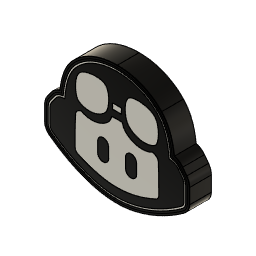
copilot-lamp (Autodesk Fusion 360 design; units mm, degrees)
Autodesk Fusion 360 part; units mm, degrees
sketch "Sketch1" plane through (0, 0, 0) normal (0, 1, 0) x (1, 0, 0)
  line L0 (0, 0) -> (250, 0)
  line L1 (250, 0) -> (250, 250)
  line L2 (250, 250) -> (0, 250)
  line L3 (0, 250) -> (0, 0)
  line L4 (10, 10) -> (240, 10)
  line L5 (240, 10) -> (240, 240)
  line L6 (240, 240) -> (10, 240)
  line L7 (10, 240) -> (10, 10)
  dimension "d1" = 250
  dimension "d2" = 250
  dimension "d3" = -10
  constraint horizontal L0
  constraint vertical L1
  constraint horizontal L2
  constraint vertical L3
  constraint coincident L0.start L3.end
  measures "d1" distance of L0.start L0.end
  measures "d2" distance of L0.start L2.end
sketch "Sketch2" plane through (0, 0, 0) normal (0, 1, 0) x (1, 0, 0)
  spline S0 degree 3 poles (158.5521, 137.3198) (158.5521, 132.1805) (154.3858, 128.0143) (149.2467, 128.0143) knots 0 0 0 0 1 1 1 1
  spline S1 degree 3 poles (149.2467, 128.0143) (144.1075, 128.0143) (139.9413, 132.1805) (139.9413, 137.3198) knots 0 0 0 0 1 1 1 1
  line L0 (139.9413, 137.3198) -> (139.9413, 154.4712)
  spline S2 degree 3 poles (139.9413, 154.4712) (139.9413, 159.6094) (144.1075, 163.7764) (149.2467, 163.7764) knots 0 0 0 0 1 1 1 1
  spline S3 degree 3 poles (149.2467, 163.7764) (154.3858, 163.7764) (158.5521, 159.6094) (158.5521, 154.4712) knots 0 0 0 0 1 1 1 1
  line L1 (158.5521, 154.4712) -> (158.5521, 137.3198)
  spline S4 degree 3 poles (101.5644, 128.0143) (106.7036, 128.0143) (110.8699, 132.1805) (110.8699, 137.3198) knots 0 0 0 0 1 1 1 1
  line L2 (110.8699, 137.3198) -> (110.8699, 154.4712)
  spline S5 degree 3 poles (110.8699, 154.4712) (110.8699, 159.6094) (106.7036, 163.7764) (101.5644, 163.7764) knots 0 0 0 0 1 1 1 1
  spline S6 degree 3 poles (101.5644, 163.7764) (96.425, 163.7764) (92.2595, 159.6094) (92.2595, 154.4712) knots 0 0 0 0 1 1 1 1
  line L3 (92.2595, 154.4712) -> (92.2595, 137.3198)
  spline S7 degree 3 poles (92.2595, 137.3198) (92.2595, 132.1805) (96.425, 128.0143) (101.5644, 128.0143) knots 0 0 0 0 1 1 1 1
  line L4 (10.7372, 128.4911) -> (10.7372, 154.1394)
  spline S8 degree 3 poles (10.7372, 154.1394) (10.7429, 157.4509) (12.3851, 160.6794) (15.0572, 162.6363) knots 0 0 0 0 1 1 1 1
  spline S9 degree 3 poles (15.0572, 162.6363) (46.6019, 185.7298) (85.5234, 204.3058) (125.1746, 204.3058) knots 0 0 0 0 1 1 1 1
  spline S10 degree 3 poles (125.1746, 204.3058) (169.0412, 204.3058) (212.9606, 179.028) (235.2919, 162.6363) knots 0 0 0 0 1 1 1 1
  spline S11 degree 3 poles (235.2919, 162.6363) (237.9639, 160.6794) (239.6054, 157.4509) (239.6119, 154.1394) knots 0 0 0 0 1 1 1 1
  line L5 (239.6119, 154.1394) -> (239.6119, 128.4911)
  spline S12 degree 3 poles (239.6119, 128.4911) (239.6119, 125.1152) (238.539, 121.8537) (236.5507, 119.1358) knots 0 0 0 0 1 1 1 1
  line L6 (236.5507, 119.1358) -> (229.5843, 109.7091)
  spline S13 degree 3 poles (229.5843, 109.7091) (225.8533, 104.6514) (220.3047, 103.3149) (214.3928, 103.3149) knots 0 0 0 0 1 1 1 1
  spline S14 degree 3 poles (214.3928, 103.3149) (212.1612, 77.8526) (206.8828, 59.6856) (194.2661, 46.3823) knots 0 0 0 0 1 1 1 1
  spline S15 degree 3 poles (194.2661, 46.3823) (170.2343, 20.92) (138.3348, 18.3452) (125.1746, 18.3452) knots 0 0 0 0 1 1 1 1
  spline S16 degree 3 poles (125.1746, 18.3452) (112.0143, 18.3452) (80.1149, 20.92) (56.083, 46.3823) knots 0 0 0 0 1 1 1 1
  spline S17 degree 3 poles (56.083, 46.3823) (43.4806, 59.6856) (38.1879, 77.8526) (35.9563, 103.3149) knots 0 0 0 0 1 1 1 1
  spline S18 degree 3 poles (35.9563, 103.3149) (30.0328, 103.3149) (24.5083, 104.6285) (20.7791, 109.7091) knots 0 0 0 0 1 1 1 1
  line L7 (20.7791, 109.7091) -> (13.8127, 119.1501)
  spline S19 degree 3 poles (13.8127, 119.1501) (11.8101, 121.868) (10.7372, 125.1152) (10.7372, 128.4911) knots 0 0 0 0 1 1 1 1
  spline S20 degree 3 poles (54.3951, 116.8328) (54.7012, 110.991) (59.4446, 108.6987) (64.3797, 107.077) knots 0 0 0 0 1 1 1 1
  spline S21 degree 3 poles (64.3797, 107.077) (69.5838, 110.3418) (75.9379, 111.6259) (82.0174, 111.6259) knots 0 0 0 0 1 1 1 1
  spline S22 degree 3 poles (82.0174, 111.6259) (88.4831, 111.6259) (100.5419, 110.081) (110.5695, 100.0677) knots 0 0 0 0 1 1 1 1
  spline S23 degree 3 poles (110.5695, 100.0677) (113.1014, 97.5501) (114.8323, 93.602) (116.0053, 89.2248) knots 0 0 0 0 1 1 1 1
  spline S24 degree 3 poles (116.0053, 89.2248) (119.0474, 88.9154) (122.1026, 88.7532) (125.1602, 88.7384) knots 0 0 0 0 1 1 1 1
  spline S25 degree 3 poles (125.1602, 88.7384) (127.8781, 88.7384) (131.0109, 88.8958) (134.3438, 89.2248) knots 0 0 0 0 1 1 1 1
  spline S26 degree 3 poles (134.3438, 89.2248) (135.5168, 93.602) (137.2477, 97.5501) (139.7796, 100.0677) knots 0 0 0 0 1 1 1 1
  spline S27 degree 3 poles (139.7796, 100.0677) (149.7929, 110.081) (161.866, 111.6259) (168.3317, 111.6259) knots 0 0 0 0 1 1 1 1
  spline S28 degree 3 poles (168.3317, 111.6259) (174.4131, 111.6259) (180.7835, 110.3561) (185.9837, 107.077) knots 0 0 0 0 1 1 1 1
  spline S29 degree 3 poles (185.9837, 107.077) (190.9031, 108.6934) (195.6269, 111.0244) (195.9397, 116.8328) knots 0 0 0 0 1 1 1 1
  spline S30 degree 3 poles (195.9397, 116.8328) (196.4636, 127.812) (196.5091, 138.7809) (196.5545, 149.755) knots 0 0 0 0 1 1 1 1
  spline S31 degree 3 poles (196.5545, 149.755) (196.5774, 155.2623) (196.6002, 160.771) (196.6836, 166.284) knots 0 0 0 0 1 1 1 1
  spline S32 degree 3 poles (196.6836, 166.284) (196.6614, 169.484) (194.7328, 172.455) (191.82, 173.7797) knots 0 0 0 0 1 1 1 1
  spline S33 degree 3 poles (191.82, 173.7797) (168.1458, 184.5654) (145.759, 190.0011) (125.1602, 190.0011) knots 0 0 0 0 1 1 1 1
  spline S34 degree 3 poles (125.1602, 190.0011) (104.5901, 190.0011) (82.2033, 184.5654) (58.5434, 173.7797) knots 0 0 0 0 1 1 1 1
  spline S35 degree 3 poles (58.5434, 173.7797) (55.631, 172.455) (53.7013, 169.484) (53.6798, 166.284) knots 0 0 0 0 1 1 1 1
  spline S36 degree 3 poles (53.6798, 166.284) (53.3966, 149.8179) (53.624, 133.2834) (54.4094, 116.8328) knots 0 0 0 0 1 1 1 1
  line L8 (54.4094, 116.8328) -> (54.3951, 116.8328)
  spline S37 degree 3 poles (191.5482, 93.8738) (187.6859, 97.7361) (180.3906, 100.3109) (172.523, 100.3109) knots 0 0 0 0 1 1 1 1
  spline S38 degree 3 poles (172.523, 100.3109) (166.515, 100.3109) (155.0713, 99.0235) (145.6302, 89.4393) knots 0 0 0 0 1 1 1 1
  spline S39 degree 3 poles (145.6302, 89.4393) (141.4819, 85.434) (138.907, 75.4208) (139.1931, 65.2645) knots 0 0 0 0 1 1 1 1
  spline S40 degree 3 poles (139.1931, 65.2645) (139.4792, 57.1108) (141.768, 50.3876) (145.2011, 47.5267) knots 0 0 0 0 1 1 1 1
  spline S41 degree 3 poles (145.2011, 47.5267) (148.9203, 44.2366) (157.3601, 42.8061) (166.8011, 43.6644) knots 0 0 0 0 1 1 1 1
  spline S42 degree 3 poles (166.8011, 43.6644) (176.8144, 44.6657) (185.2541, 47.9558) (189.5455, 52.5333) knots 0 0 0 0 1 1 1 1
  spline S43 degree 3 poles (189.5455, 52.5333) (198.8436, 62.6896) (196.8409, 88.438) (191.5482, 93.8738) knots 0 0 0 0 1 1 1 1
  spline S44 degree 3 poles (133.1852, 68.8406) (132.8991, 70.4141) (132.756, 72.1307) (132.613, 73.9903) knots 0 0 0 0 1 1 1 1
  spline S45 degree 3 poles (132.613, 73.9903) (132.613, 75.2777) (132.613, 76.5651) (132.756, 77.9956) knots 0 0 0 0 1 1 1 1
  spline S46 degree 3 poles (132.756, 77.9956) (129.8951, 77.7095) (127.4633, 77.7095) (125.1746, 77.7095) knots 0 0 0 0 1 1 1 1
  spline S47 degree 3 poles (125.1746, 77.7095) (122.8861, 77.7095) (120.454, 77.7095) (117.5931, 77.9956) knots 0 0 0 0 1 1 1 1
  spline S48 degree 3 poles (117.5931, 77.9956) (117.7361, 76.5651) (117.7361, 75.278) (117.7361, 73.9906) knots 0 0 0 0 1 1 1 1
  spline S49 degree 3 poles (117.7361, 73.9906) (117.5931, 72.131) (117.45, 70.4141) (117.1639, 68.8406) knots 0 0 0 0 1 1 1 1
  spline S50 degree 3 poles (117.1639, 68.8406) (120.1679, 68.5545) (122.8858, 68.4115) (125.1746, 68.4115) knots 0 0 0 0 1 1 1 1
  spline S51 degree 3 poles (125.1746, 68.4115) (127.4633, 68.4115) (130.1812, 68.5545) (133.1852, 68.8406) knots 0 0 0 0 1 1 1 1
  spline S52 degree 3 poles (111.156, 65.2645) (111.4421, 75.4208) (108.8672, 85.434) (104.7189, 89.4393) knots 0 0 0 0 1 1 1 1
  spline S53 degree 3 poles (104.7189, 89.4393) (95.2778, 99.0235) (83.8341, 100.3109) (77.8261, 100.3109) knots 0 0 0 0 1 1 1 1
  spline S54 degree 3 poles (77.8261, 100.3109) (69.9585, 100.3109) (62.6632, 97.7361) (58.8009, 93.8738) knots 0 0 0 0 1 1 1 1
  spline S55 degree 3 poles (58.8009, 93.8738) (53.5082, 88.438) (51.5055, 62.6896) (60.8036, 52.5333) knots 0 0 0 0 1 1 1 1
  spline S56 degree 3 poles (60.8036, 52.5333) (65.095, 47.9558) (73.5347, 44.6657) (83.548, 43.6644) knots 0 0 0 0 1 1 1 1
  spline S57 degree 3 poles (83.548, 43.6644) (92.9891, 42.8061) (101.4288, 44.2366) (105.148, 47.5267) knots 0 0 0 0 1 1 1 1
  spline S58 degree 3 poles (105.148, 47.5267) (108.5811, 50.3876) (110.8699, 57.1108) (111.156, 65.2645) knots 0 0 0 0 1 1 1 1
  line L9 (7.7372, 128.4911) -> (7.7372, 154.1445)
  spline S59 degree 3 poles (7.7372, 154.1445) (7.7441, 158.1057) (9.5073, 161.8673) (12.4918, 164.4276) (12.747, 164.6466) (13.0114, 164.8566) (13.2847, 165.0567) (13.2848, 165.0567) (13.2848, 165.0568) (13.2849, 165.0568) knots 0 0 0 0 0.921211 0.921211 0.921211 1 1 1 1.000024 1.000024 1.000024 1.000024
  spline S60 degree 3 poles (13.2849, 165.0568) (13.285, 165.0569) (13.285, 165.0569) (13.2851, 165.057) (38.021, 183.1658) (67.2869, 198.586) (98.1418, 204.6126) (107.0469, 206.352) (116.084, 207.3058) (125.1746, 207.3058) knots -0.000002 -0.000002 -0.000002 -0.000002 0 0 0 0.776029 0.776029 0.776029 1 1 1 1
  spline S61 degree 3 poles (125.1746, 207.3058) (151.1392, 207.3058) (176.8345, 198.726) (198.2832, 188.335) (214.0222, 180.7101) (227.4746, 172.0956) (237.0644, 165.0567) knots 0 0 0 0 0.576746 0.576746 0.576746 0.999961 0.999961 0.999961 0.999961
  spline S62 degree 3 poles (237.0644, 165.0567) (240.2611, 162.7155) (242.2626, 159.0731) (242.5713, 155.1511) (242.5975, 154.8176) (242.6112, 154.4821) (242.6119, 154.1452) (242.6119, 154.1442) (242.6119, 154.1433) (242.6119, 154.1423) knots 0 0 0 0 0.92164 0.92164 0.92164 1 1 1 1.000295 1.000295 1.000295 1.000295
  line L10 (242.6119, 154.1423) -> (242.6119, 128.4911)
  spline S63 degree 3 poles (242.6119, 128.4911) (242.6119, 124.4796) (241.3319, 120.5904) (238.9719, 117.3645) (238.9705, 117.3626) (238.9691, 117.3606) (238.9677, 117.3587) knots 0 0 0 0 1 1 1 1.000715 1.000715 1.000715 1.000715
  line L11 (238.9677, 117.3587) -> (231.9977, 107.9271)
  spline S64 degree 3 poles (231.9977, 107.9271) (229.8034, 104.953) (226.9585, 102.9755) (223.9284, 101.8321) (221.7257, 101.0009) (219.4347, 100.5852) (217.1364, 100.413) knots 0.000057 0.000057 0.000057 0.000057 0.495955 0.495955 0.495955 0.856432 0.856432 0.856432 0.856432
  spline S65 degree 3 poles (217.1364, 100.413) (215.652, 85.2695) (213.0029, 72.5806) (208.1192, 61.8381) (205.1344, 55.2727) (201.3057, 49.4466) (196.4478, 44.3231) knots 0.034498 0.034498 0.034498 0.034498 0.633678 0.633678 0.633678 0.999875 0.999875 0.999875 0.999875
  spline S66 degree 3 poles (196.4478, 44.3232) (182.9181, 29.9881) (166.9642, 22.6605) (153.1177, 18.9787) (141.5097, 15.8921) (131.3545, 15.3452) (125.1746, 15.3452) knots 0 0 0 0 0.543971 0.543971 0.543971 1 1 1 1
  spline S67 degree 3 poles (125.1746, 15.3452) (116.3753, 15.3452) (99.5093, 16.4426) (81.8828, 24.4301) (72.3644, 28.7433) (62.6264, 35.0798) (53.9051, 44.3191) knots 0 0 0 0 0.649314 0.649314 0.649314 0.999949 0.999949 0.999949 0.999949
  spline S68 degree 3 poles (53.9051, 44.3191) (46.3224, 52.3236) (41.2686, 62.0288) (37.9494, 73.6262) (35.6681, 81.5973) (34.1875, 90.4726) (33.2128, 100.4115) knots 0 0 0 0 0.572201 0.572201 0.572201 0.965484 0.965484 0.965484 0.965484
  spline S69 degree 3 poles (33.2128, 100.4115) (30.5434, 100.609) (27.8843, 101.1321) (25.3703, 102.2565) (22.7389, 103.4334) (20.2964, 105.2967) (18.3607, 107.9339) knots 0.143547 0.143547 0.143547 0.143547 0.562009 0.562009 0.562009 1 1 1 1
  line L12 (18.3607, 107.9339) -> (11.3976, 117.3705)
  spline S70 degree 3 poles (11.3976, 117.3705) (9.0215, 120.5952) (7.7372, 124.4796) (7.7372, 128.4911) knots 0 0 0 0 1 1 1 1
  spline S71 degree 3 poles (8.9824, 115.5909) (6.233, 119.3223) (4.7372, 123.844) (4.7372, 128.4911) knots 0 0 0 0 1 1 1 1
  line L13 (4.7372, 128.4911) -> (4.7372, 154.1445)
  spline S72 degree 3 poles (4.7372, 154.1445) (4.7372, 154.1463) (4.7372, 154.148) (4.7372, 154.1497) (4.7442, 158.1771) (6.2198, 161.9705) (8.7807, 164.9481) (9.5825, 165.8803) (10.4953, 166.7323) (11.5122, 167.4771) (11.5123, 167.4772) (11.5125, 167.4772) (11.5126, 167.4773) knots -0.000521 -0.000521 -0.000521 -0.000521 0 0 0 0.761555 0.761555 0.761555 1 1 1 1.000048 1.000048 1.000048 1.000048
  spline S73 degree 3 poles (11.5126, 167.4773) (11.5127, 167.4774) (11.5128, 167.4775) (11.513, 167.4776) (32.5289, 182.8631) (56.8066, 196.3546) (82.7045, 203.9271) (96.4932, 207.9589) (110.7471, 210.3058) (125.1746, 210.3058) knots -0.000004 -0.000004 -0.000004 -0.000004 0 0 0 0.65256 0.65256 0.65256 1 1 1 1
  spline S74 degree 3 poles (125.1746, 210.3058) (146.7387, 210.3058) (167.9411, 204.5481) (186.7543, 196.7918) (208.2194, 187.9422) (226.5873, 176.468) (238.837, 167.477) knots 0 0 0 0 0.467044 0.467044 0.467044 0.999924 0.999924 0.999924 0.999924
  spline S75 degree 3 poles (238.837, 167.477) (242.0897, 165.0948) (244.2873, 161.6622) (245.1818, 157.8319) (245.4602, 156.6399) (245.6094, 155.4058) (245.6119, 154.1511) (245.6119, 154.1491) (245.6119, 154.1472) (245.6119, 154.1452) knots 0 0 0 0 0.762657 0.762657 0.762657 1 1 1 1.000589 1.000589 1.000589 1.000589
  line L14 (245.6119, 154.1452) -> (245.6119, 128.4911)
  spline S76 degree 3 poles (245.6119, 128.4911) (245.6119, 123.844) (244.1248, 119.3271) (241.3932, 115.5932) (241.3903, 115.5893) (241.3875, 115.5854) (241.3846, 115.5815) knots 0 0 0 0 1 1 1 1.001431 1.001431 1.001431 1.001431
  line L15 (241.3846, 115.5815) -> (234.4112, 106.1452)
  spline S77 degree 3 poles (234.4112, 106.1452) (232.3088, 103.2959) (229.6221, 101.1651) (226.7745, 99.7909) (224.5136, 98.6997) (222.1772, 98.0622) (219.8733, 97.7062) knots 0.000099 0.000099 0.000099 0.000099 0.410804 0.410804 0.410804 0.736901 0.736901 0.736901 0.736901
  spline S78 degree 3 poles (219.8733, 97.7062) (218.6013, 85.9602) (216.5742, 75.613) (213.2182, 66.4036) (209.8594, 57.1866) (205.124, 49.1134) (198.6246, 42.2588) knots 0.066215 0.066215 0.066215 0.066215 0.532858 0.532858 0.532858 0.99988 0.99988 0.99988 0.99988
  spline S79 degree 3 poles (198.6246, 42.2588) (187.2956, 30.2574) (174.2956, 22.9932) (162.2131, 18.6679) (146.8735, 13.1765) (132.9735, 12.3452) (125.1746, 12.3452) knots 0.000064 0.000064 0.000064 0.000064 0.440648 0.440648 0.440648 1 1 1 1
  spline S80 degree 3 poles (125.1746, 12.3452) (117.5616, 12.3452) (104.1361, 13.1384) (89.2315, 18.2828) (77.5633, 22.31) (64.9648, 29.0431) (53.7854, 40.1449) (53.0936, 40.8319) (52.4073, 41.5355) (51.7272, 42.256) knots 0 0 0 0 0.546006 0.546006 0.546006 0.97345 0.97345 0.97345 0.999902 0.999902 0.999902 0.999902
  line L16 (51.7272, 42.256) -> (51.7196, 42.264)
  spline S81 degree 3 poles (51.7196, 42.264) (45.1771, 49.1727) (40.4206, 57.3182) (37.0555, 66.6268) (33.7472, 75.7787) (31.739, 86.0521) (30.4764, 97.7022) knots 0.000182 0.000182 0.000182 0.000182 0.470924 0.470924 0.470924 0.933737 0.933737 0.933737 0.933737
  spline S82 degree 3 poles (30.4764, 97.7022) (28.8084, 97.9581) (27.1205, 98.3623) (25.4513, 98.9838) (22.5741, 100.0551) (19.7525, 101.8165) (17.4328, 104.3431) (16.9117, 104.9107) (16.4155, 105.5144) (15.947, 106.1522) knots 0.26327 0.26327 0.26327 0.26327 0.5 0.5 0.5 0.908036 0.908036 0.908036 0.999687 0.999687 0.999687 0.999687
  line L17 (15.947, 106.1522) -> (8.9824, 115.5909)
  line L18 (1.7372, 128.4911) -> (1.7372, 154.1471)
  spline S83 degree 3 poles (1.7372, 154.1471) (1.7372, 154.1497) (1.7372, 154.1523) (1.7372, 154.1549) (1.7445, 158.3641) (3.1041, 162.3187) (5.4807, 165.605) (6.6481, 167.2193) (8.0725, 168.6765) (9.7397, 169.8974) (9.7399, 169.8976) (9.7401, 169.8977) (9.7403, 169.8979) knots -0.000782 -0.000782 -0.000782 -0.000782 0 0 0 0.67059 0.67059 0.67059 1 1 1 1.000072 1.000072 1.000072 1.000072
  spline S84 degree 3 poles (9.7403, 169.8979) (9.7405, 169.898) (9.7407, 169.8981) (9.7408, 169.8983) (28.9256, 183.9432) (50.8226, 196.4464) (74.2971, 204.4158) (90.6333, 209.9618) (107.7504, 213.3058) (125.1746, 213.3058) knots -0.000006 -0.000006 -0.000006 -0.000006 0 0 0 0.589654 0.589654 0.589654 1 1 1 1
  spline S85 degree 3 poles (125.1746, 213.3058) (144.9594, 213.3058) (164.3076, 208.5849) (181.8206, 201.9667) (203.0931, 193.9278) (221.6874, 183.0627) (235.0889, 173.8226) (237.0417, 172.4762) (238.8843, 171.1636) (240.6095, 169.8974) knots 0 0 0 0 0.418071 0.418071 0.418071 0.925892 0.925892 0.925892 0.999887 0.999887 0.999887 0.999887
  spline S86 degree 3 poles (240.6095, 169.8973) (244.0092, 167.4076) (246.4055, 163.9735) (247.659, 160.1093) (248.2717, 158.2204) (248.6078, 156.217) (248.6119, 154.1569) (248.6119, 154.154) (248.6119, 154.1511) (248.6119, 154.1481) knots 0 0 0 0 0.671667 0.671667 0.671667 1 1 1 1.000884 1.000884 1.000884 1.000884
  line L19 (248.6119, 154.1481) -> (248.6119, 128.4911)
  spline S87 degree 3 poles (248.6119, 128.4911) (248.6119, 123.2084) (246.9177, 118.0638) (243.8144, 113.8219) (243.8101, 113.816) (243.8059, 113.8102) (243.8016, 113.8044) knots 0 0 0 0 1 1 1 1.002146 1.002146 1.002146 1.002146
  line L20 (243.8016, 113.8044) -> (236.8246, 104.3632)
  spline S88 degree 3 poles (236.8246, 104.3632) (234.6676, 101.4402) (231.9233, 99.1301) (229.0143, 97.566) (226.9061, 96.4327) (224.7352, 95.6748) (222.6063, 95.1795) knots 0.00013 0.00013 0.00013 0.00013 0.371204 0.371204 0.371204 0.64011 0.64011 0.64011 0.64011
  spline S89 degree 3 poles (222.6063, 95.1795) (221.4019, 84.9995) (219.5897, 75.8015) (216.7493, 67.405) (213.7871, 58.6485) (209.6663, 50.7578) (204.052, 43.886) (203.0185, 42.6209) (201.9358, 41.391) (200.8039, 40.1971) knots 0.09523 0.09523 0.09523 0.09523 0.5 0.5 0.5 0.92212 0.92212 0.92212 0.999827 0.999827 0.999827 0.999827
  spline S90 degree 3 poles (200.8039, 40.1971) (190.3969, 29.173) (178.6023, 22.0055) (167.376, 17.4311) (150.9666, 10.7448) (135.7546, 9.4848) (126.7582, 9.3565) (126.2065, 9.3486) (125.6782, 9.3452) (125.1746, 9.3452) knots 0.000092 0.000092 0.000092 0.000092 0.392007 0.392007 0.392007 0.964867 0.964867 0.964867 1 1 1 1
  spline S91 degree 3 poles (125.1746, 9.3452) (118.0074, 9.3452) (105.873, 10.026) (92.0949, 14.2023) (81.2926, 17.4767) (69.4489, 22.9307) (58.4185, 31.9369) (55.3818, 34.4163) (52.4092, 37.1631) (49.5435, 40.1989) knots 0 0 0 0 0.5 0.5 0.5 0.892007 0.892007 0.892007 0.999929 0.999929 0.999929 0.999929
  spline S92 degree 3 poles (49.5435, 40.1989) (43.3927, 46.6934) (38.7397, 54.2543) (35.3445, 62.6963) (31.4756, 72.3165) (29.179, 83.0561) (27.7439, 95.1732) knots 0.000132 0.000132 0.000132 0.000132 0.422915 0.422915 0.422915 0.904698 0.904698 0.904698 0.904698
  spline S93 degree 3 poles (27.7439, 95.1732) (27.057, 95.3324) (26.3631, 95.5197) (25.6684, 95.7386) (22.6905, 96.6768) (19.651, 98.2413) (17.0091, 100.5649) (15.7415, 101.6797) (14.5706, 102.959) (13.5312, 104.3735) knots 0.360177 0.360177 0.360177 0.360177 0.447249 0.447249 0.447249 0.820486 0.820486 0.820486 0.999574 0.999574 0.999574 0.999574
  line L21 (13.5312, 104.3735) -> (6.5672, 113.8113)
  spline S94 degree 3 poles (6.5672, 113.8113) (3.4444, 118.0494) (1.7372, 123.2084) (1.7372, 128.4911) knots 0 0 0 0 1 1 1 1
  dimension "d4" = -3
  dimension "d5" = -6
  dimension "d6" = -9
extrude "Extrude1" add sketch "Sketch2" along normal blind 2 from surface at 36 contours S0 S1 L0 S2 S3 L1 | S4 L2 S5 S6 L3 S7 | L4 S8 S9 S10 S11 L5 S12 L6 S13 S14 S15 S16 S17 S18 L7 S19 | S20 S21 S22 S23 S24 S25 S26 S27 S28 S29 S30 S31 S32 S33 S34 S35 S36 L8 | S37 S38 S39 S40 S41 S42 S43 | S44 S45 S46 S47 S48 S49 S50 S51 | S52 S53 S54 S55 S56 S57 S58 | L9 S59 S60 S61 S62 L10 S63 L11 S64 S65 S66 S67 S68 S69 L12 S70 | S71 L13 S72 S73 S74 S75 L14 S76 L15 S77 S78 S79 S80 L16 S81 S82 L17 | L18 S83 S84 S85 S86 L19 S87 L20 S88 S89 S90 S91 S92 S93 L21 S94 makes body 1 in component "Back"
extrude "Extrude2" add sketch "Sketch2" along normal blind 36 contours L18 S83 S84 S85 S86 L19 S87 L20 S88 S89 S90 S91 S92 S93 L21 S94 bodies 1 in component "Back"
extrude "Extrude1'" add sketch "Sketch2" along normal blind 1 separate body contours S0 S1 L0 S2 S3 L1 | S4 L2 S5 S6 L3 S7 | L4 S8 S9 S10 S11 L5 S12 L6 S13 S14 S15 S16 S17 S18 L7 S19 | S71 L13 S72 S73 S74 S75 L14 S76 L15 S77 S78 S79 S80 L16 S81 S82 L17 | L18 S83 S84 S85 S86 L19 S87 L20 S88 S89 S90 S91 S92 S93 L21 S94 makes body 2 at (39.604, 0, -145.752) makes body 3 at (104.6664, 0, -143.0369) makes body 4 at (59.3296, 0, -193.8677) makes body 5 at (152.3485, 0, -143.0369) in component "Black"
extrude "Extrude2'" add sketch "Sketch2" along normal blind 5 contours S71 L13 S72 S73 S74 S75 L14 S76 L15 S77 S78 S79 S80 L16 S81 S82 L17 bodies 4 in component "Black"
extrude "Extrude1''" add sketch "Sketch2" along normal blind 0.6 separate body contours S20 S21 S22 S23 S24 S25 S26 S27 S28 S29 S30 S31 S32 S33 S34 S35 S36 L8 | S37 S38 S39 S40 S41 S42 S43 | S44 S45 S46 S47 S48 S49 S50 S51 | S52 S53 S54 S55 S56 S57 S58 | L9 S59 S60 S61 S62 L10 S63 L11 S64 S65 S66 S67 S68 S69 L12 S70 makes body 6 at (127.654, 0, -73.3704) makes body 7 at (73.6219, 0, -71.4895) makes body 8 at (66.7829, 0, -140.1455) makes body 9 at (214.1719, 0, -94.6407) makes body 10 at (175.5613, 0, -70.1364) in component "White"
sketch "Sketch5" plane through (0, 0, 0) normal (0, 0, 1) x (1, 0, 0)
  line L0 (140.7612, 34.7806, -209.7825) -> (109.4367, 34.7806, -209.7825)
  line L1 (109.4367, 34.7806, -209.7825) -> (109.4367, 26.6706, -209.7825)
  line L2 (109.4367, 26.6706, -209.7825) -> (140.7612, 26.6706, -209.7825)
  line L3 (140.7612, 26.6706, -209.7825) -> (140.7612, 34.7806, -209.7825)
extrude "Extrude3" cut sketch "Sketch5" against normal blind 10 contours L0 L1 L2 L3 in plane through (0, 0, -209.7825) normal (0, 0, 1) bodies 1 in component "Back"
extrude "Extrude4" add sketch "Sketch2" against normal blind 10 from surface at 36 contours S71 L13 S72 S73 S74 S75 L14 S76 L15 S77 S78 S79 S80 L16 S81 S82 L17 bodies 1 in component "Back"
extrude "Extrude5" cut sketch "Sketch5" along normal blind 30 contours L0 L1 L2 L3 in plane through (0, 0, -209.7825) normal (0, 0, 1) bodies 1 in component "Back"
extrude "Extrude6" cut sketch "Sketch5" against normal blind 16 contours L0 L1 L2 L3 in plane through (0, 0, -209.7825) normal (0, 0, 1) bodies 1 in component "Back"
sketch "Sketch6" plane through (0, 27, 0) normal (0, -1, 0) x (1, 0, 0)
  spline S0 degree 3 poles (30.4764, -97.7022) (28.8084, -97.9581) (27.1205, -98.3623) (25.4513, -98.9838) (22.5741, -100.0551) (19.7525, -101.8165) (17.4328, -104.3431) (16.9117, -104.9107) (16.4155, -105.5144) (15.947, -106.1522) knots 0.26327 0.26327 0.26327 0.26327 0.5 0.5 0.5 0.908036 0.908036 0.908036 0.999687 0.999687 0.999687 0.999687
  line L0 (15.947, -106.1522) -> (8.9824, -115.5909)
  spline S1 degree 3 poles (8.9824, -115.5909) (6.233, -119.3223) (4.7372, -123.844) (4.7372, -128.4911) knots 0 0 0 0 1 1 1 1
  line L1 (4.7372, -128.4911) -> (4.7372, -154.1445)
  spline S2 degree 3 poles (4.7372, -154.1445) (4.7372, -154.1463) (4.7372, -154.148) (4.7372, -154.1497) (4.7442, -158.1771) (6.2198, -161.9705) (8.7807, -164.9481) (9.5825, -165.8803) (10.4953, -166.7323) (11.5122, -167.4771) (11.5123, -167.4772) (11.5125, -167.4772) (11.5126, -167.4773) knots -0.000521 -0.000521 -0.000521 -0.000521 0 0 0 0.761555 0.761555 0.761555 1 1 1 1.000048 1.000048 1.000048 1.000048
  spline S3 degree 3 poles (11.5126, -167.4773) (11.5127, -167.4774) (11.5128, -167.4775) (11.513, -167.4776) (32.5289, -182.8631) (56.8066, -196.3546) (82.7045, -203.9271) (96.4932, -207.9589) (110.7471, -210.3058) (125.1746, -210.3058) knots -0.000004 -0.000004 -0.000004 -0.000004 0 0 0 0.65256 0.65256 0.65256 1 1 1 1
  spline S4 degree 3 poles (125.1746, -210.3058) (146.7387, -210.3058) (167.9411, -204.5481) (186.7543, -196.7918) (208.2194, -187.9422) (226.5873, -176.468) (238.837, -167.477) knots 0 0 0 0 0.467044 0.467044 0.467044 0.999924 0.999924 0.999924 0.999924
  spline S5 degree 3 poles (238.837, -167.477) (242.0897, -165.0948) (244.2873, -161.6622) (245.1818, -157.8319) (245.4602, -156.6399) (245.6094, -155.4058) (245.6119, -154.1511) (245.6119, -154.1491) (245.6119, -154.1472) (245.6119, -154.1452) knots 0 0 0 0 0.762657 0.762657 0.762657 1 1 1 1.000589 1.000589 1.000589 1.000589
  line L2 (245.6119, -154.1452) -> (245.6119, -128.4911)
  spline S6 degree 3 poles (245.6119, -128.4911) (245.6119, -123.844) (244.1248, -119.3271) (241.3932, -115.5932) (241.3903, -115.5893) (241.3875, -115.5854) (241.3846, -115.5815) knots 0 0 0 0 1 1 1 1.001431 1.001431 1.001431 1.001431
  line L3 (241.3846, -115.5815) -> (234.4112, -106.1452)
  spline S7 degree 3 poles (234.4112, -106.1452) (232.3088, -103.2959) (229.6221, -101.1651) (226.7745, -99.7909) (224.5136, -98.6997) (222.1772, -98.0622) (219.8733, -97.7062) knots 0.000099 0.000099 0.000099 0.000099 0.410804 0.410804 0.410804 0.736901 0.736901 0.736901 0.736901
  spline S8 degree 3 poles (219.8733, -97.7062) (218.6013, -85.9602) (216.5742, -75.613) (213.2182, -66.4036) (209.8594, -57.1866) (205.124, -49.1134) (198.6246, -42.2588) knots 0.066215 0.066215 0.066215 0.066215 0.532858 0.532858 0.532858 0.99988 0.99988 0.99988 0.99988
  spline S9 degree 3 poles (198.6246, -42.2588) (187.2956, -30.2574) (174.2956, -22.9932) (162.2131, -18.6679) (146.8735, -13.1765) (132.9735, -12.3452) (125.1746, -12.3452) knots 0.000064 0.000064 0.000064 0.000064 0.440648 0.440648 0.440648 1 1 1 1
  spline S10 degree 3 poles (125.1746, -12.3452) (117.5616, -12.3452) (104.1361, -13.1384) (89.2315, -18.2828) (77.5633, -22.31) (64.9648, -29.0431) (53.7854, -40.1449) (53.0936, -40.8319) (52.4073, -41.5355) (51.7272, -42.256) knots 0 0 0 0 0.546006 0.546006 0.546006 0.97345 0.97345 0.97345 0.999902 0.999902 0.999902 0.999902
  line L4 (51.7272, -42.256) -> (51.7196, -42.264)
  spline S11 degree 3 poles (51.7196, -42.264) (45.1771, -49.1727) (40.4206, -57.3182) (37.0555, -66.6268) (33.7472, -75.7787) (31.739, -86.0521) (30.4764, -97.7022) knots 0.000182 0.000182 0.000182 0.000182 0.470924 0.470924 0.470924 0.933737 0.933737 0.933737 0.933737
  line L5 (109.4643, -212.8898) -> (140.6907, -212.8898)
  line L6 (140.6907, -212.8898) -> (140.6907, -199.7734)
  line L7 (140.6907, -199.7734) -> (109.4643, -199.7734)
  line L8 (109.4643, -199.7734) -> (109.4643, -212.8898)
  constraint horizontal L5
  constraint vertical L6
  constraint horizontal L7
  constraint vertical L8
extrude "Extrude7" add sketch "Sketch2" against normal blind 10 from surface at 36 contours L9 S59 S60 S61 S62 L10 S63 L11 S64 S65 S66 S67 S68 S69 L12 S70 bodies 1 in component "Back"
extrude "Extrude1'''" add sketch "Sketch2" along normal blind 1 from surface at 26 separate body contours S0 S1 L0 S2 S3 L1 | S4 L2 S5 S6 L3 S7 | L4 S8 S9 S10 S11 L5 S12 L6 S13 S14 S15 S16 S17 S18 L7 S19 | S20 S21 S22 S23 S24 S25 S26 S27 S28 S29 S30 S31 S32 S33 S34 S35 S36 L8 | S37 S38 S39 S40 S41 S42 S43 | S44 S45 S46 S47 S48 S49 S50 S51 | S52 S53 S54 S55 S56 S57 S58 | L9 S59 S60 S61 S62 L10 S63 L11 S64 S65 S66 S67 S68 S69 L12 S70 makes body 11 in component "Reflector"
extrude "Extrude2''" cut sketch "Sketch6" along normal blind 6 contours S3 S4 L6 L7 L8 bodies 11 in component "Reflector"
extrude "Extrude8" cut sketch "Sketch2" along normal blind 1 from surface at 26 contours L9 S59 S60 S61 S62 L10 S63 L11 S64 S65 S66 S67 S68 S69 L12 S70 bodies 1 in component "Back"
extrude "Extrude9" cut sketch "Sketch5" along normal blind 12 contours L0 L1 L2 L3 in plane through (0, 0, -209.7825) normal (0, 0, 1) bodies 1 in component "Back"
extrude "Extrude10" cut sketch "Sketch6" along normal blind 5 contours S3 S4 L6 L7 L8 bodies 1 in component "Back"
component "Back" placed x (1, 0, 0) y (0, 1, 0) z (0, 0, 1) at (0, 0, 0)
component "Black" placed x (1, 0, 0) y (0, 1, 0) z (0, 0, 1) at (0, 0, 0)
component "White" placed x (1, 0, 0) y (0, 1, 0) z (0, 0, 1) at (0, 0, 0)
component "Reflector" placed x (1, 0, 0) y (0, 1, 0) z (0, 0, 1) at (0, 0, 0)
